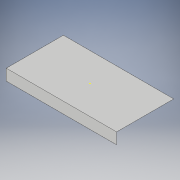
# Autodesk Inventor part: Gehaeuse_Deckel
Saved by Autodesk Inventor 2019 (Build 230136000, 136)
## iProperties
Created: 2019-01-15
Part Number: Gehaeuse_Deckel
Material: Generic
Document SubType Name: Modeling
Designer: patri
Density: 1 g/cm^3
Appearance: Default
Author: patri
Autodesk Inventor part; units mm, degrees
ref_plane "YZ Plane" through (0, 0, 0) normal (1, 0, 0) x (0, 1, 0)
ref_plane "XZ Plane" through (0, 0, 0) normal (0, 1, 0) x (-1, 0, 0)
ref_plane "XY Plane" through (0, 0, 0) normal (0, 0, 1) x (1, 0, 0)
sketch "Sketch1" plane through (0, 0, 0) normal (0, 1, 0) x (-1, 0, 0)
  line L0 (222, -115) -> (-222, -115)
  line L1 (-222, -115) -> (-222, 115)
  line L2 (-222, 115) -> (222, 115)
  line L3 (222, 115) -> (222, -115)
  line L4 (0, -161) -> (0, 161) projected
  line L5 (310.8, 0) -> (-310.8, 0) projected
  point P0 (0, 0)
  dimension "d0" = 444
  dimension "d1" = 230
  constraints: 8 end point, 2 parallel, 1 horizontal, 1 perpendicular, 2 other
  measures "d0" distance of L0.start L0.end
  measures "d1" distance of L0.end L1.end
extrude "Extrusion1" add sketch "Sketch1" along normal blind 0.12
sketch "Sketch2" plane through (0, 0.12, 0) normal (0, 1, 0) x (1, 0, 0)
  point P0 (0, 0)
sketch "Sketch4" plane through (-222, 0, 115) normal (0, 0, 1) x (1, 0, 0)
  line L0 (444, 0.12) -> (0, 0.12) projected
  line L1 (0, 0.12) -> (444, 0.12)
  line L2 (444, 0.12) -> (444, -44.88)
  line L3 (444, -44.88) -> (0, -44.88)
  line L4 (0, -44.88) -> (0, 0.12)
  point P0 (222, 0)
  dimension "d4" = 444
  dimension "d5" = 45
  constraints: 8 end point, 2 parallel, 1 horizontal, 1 perpendicular
  measures "d4" distance of L2.end L3.end
  measures "d5" distance of L1.end L2.end
extrude "Extrusion2" add sketch "Sketch4" against normal blind 0.12
body "Solid1"
